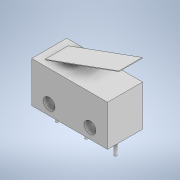
# Autodesk Inventor part: Micro Switch
Saved by Autodesk Inventor 2021 (Build 250183000, 183)
## iProperties
Created: 2021-08-25
Part Number: Micro Switch
Material: Genérico
Document SubType Name: Modeling
Designer: Diego.labarca
Density: 1 g/cm^3
Appearance: Valor por defecto
Author: Diego.labarca
Autodesk Inventor part; units mm, degrees
ref_plane "YZ Plane" through (0, 0, 0) normal (1, 0, 0) x (0, 1, 0)
ref_plane "XZ Plane" through (0, 0, 0) normal (0, 1, 0) x (-1, 0, 0)
ref_plane "XY Plane" through (0, 0, 0) normal (0, 0, 1) x (1, 0, 0)
sketch "Boceto1" plane through (0, 0, 0) normal (0, 0, 1) x (1, 0, 0)
  line L0 (-6.5, 3.5) -> (6.5, 3.5)
  line L1 (6.5, 3.5) -> (6.5, -3.5)
  line L2 (6.5, -3.5) -> (-6.5, -3.5)
  line L3 (-6.5, -3.5) -> (-6.5, 3.5)
  line L4 (0, -4.9) -> (0, 4.9) projected
  line L5 (-9.1, 0) -> (9.1, 0) projected
  point P0 (0, 0)
  dimension "d0" = 13
  dimension "d1" = 7
  constraints: 8 end point, 2 parallel, 1 horizontal, 1 perpendicular, 2 other
  measures "d0" distance of L1.end L2.end
  measures "d1" distance of L0.end L1.end
extrude "Extrusión1" add sketch "Boceto1" along normal mid plane 6
sketch "Boceto2" plane through (0, 0, 3) normal (0, 0, 1) x (1, 0, 0)
  circle A0 centre (3.5, -1.75) radius 1
  circle A1 centre (-3.5, -1.75) radius 1
  line L0 (-6.5, 3.5) -> (-6.5, -3.5) projected
  line L1 (6.5, -3.5) -> (6.5, 3.5) projected
  line L2 (-6.5, -3.5) -> (6.5, -3.5) projected
  point P0 (0, 0)
  dimension "d4" = 2
  dimension "d5" = 2
  dimension "d6" = 3
  dimension "d8" = 3
  dimension "d25" = 1.75
  dimension "d26" = 1.75
  constraints: 2 centre point
  measures "d4" diameter of A0
  measures "d5" diameter of A1
  measures "d6" distance from line of L0 A1.centre
  measures "d8" distance from line of L1 A0.centre
  measures "d25" distance from line of L2 A0.centre
  measures "d26" distance from line of L2 A1.centre
extrude "Extrusión2" cut sketch "Boceto2" against normal up to surface (6 mm away)
sketch "Boceto3" plane through (0, 0, 0) normal (0, 0, 1) x (1, 0, 0)
  line L0 (-6.5, 3.5) -> (6.5, 3.5) projected
  line L1 (-6.5, 3.5) -> (-5.25, 3.5)
  line L2 (-5.25, 3.5) -> (7.4359, 8.1173)
  line L3 (7.4359, 8.1173) -> (7.4701, 8.0233)
  line L4 (7.4701, 8.0233) -> (-4.9576, 3.5)
  line L5 (-4.9576, 3.5) -> (-5.25, 3.5)
  point P0 (0, 0)
  dimension "d11" = 1.25
  dimension "d12" = 13.5
  dimension "d13" = 160
  dimension "d14" = 0.1
  dimension "d15" = 90
  constraints: 10 end point, 2 point on line, 1 collinear, 1 perpendicular
  measures "d11" distance of L0.start L1.end
  measures "d12" distance of L1.end L2.end
  measures "d13" angle of L2 L1
  measures "d14" distance of L2.end L3.end
  measures "d15" angle of L3 L4
extrude "Extrusión3" add sketch "Boceto3" against normal mid plane 4
sketch "Boceto4" plane through (-6.5, -3.5, -3) normal (0, -1, 0) x (1, 0, 0)
  circle A0 centre (1.5, 3.1423) radius 0.25
  circle A1 centre (11.5, 3.1423) radius 0.25
  line L0 (0, 0) -> (0, 6) projected
  circle A2 centre (6.5, 3.1423) radius 0.25
  line L1 (13, 6) -> (13, 0) projected
  point P0 (6.5, 3)
  dimension "d18" = 1.5
  dimension "d20" = 0.5
  dimension "d21" = 0.5
  dimension "d22" = 0.5
  dimension "d27" = 1.5
  constraints: 3 centre point
  measures "d18" distance from line of L0 A0.centre
  measures "d20" diameter of A0
  measures "d21" diameter of A2
  measures "d22" diameter of A1
  measures "d27" distance from line of L1 A1.centre
extrude "Extrusión4" add sketch "Boceto4" along normal blind 3
equation "\"d5\" = d4"
equation "\"d26\" = d25"
equation "\"d21\" = d20"
equation "\"d22\" = d21"
